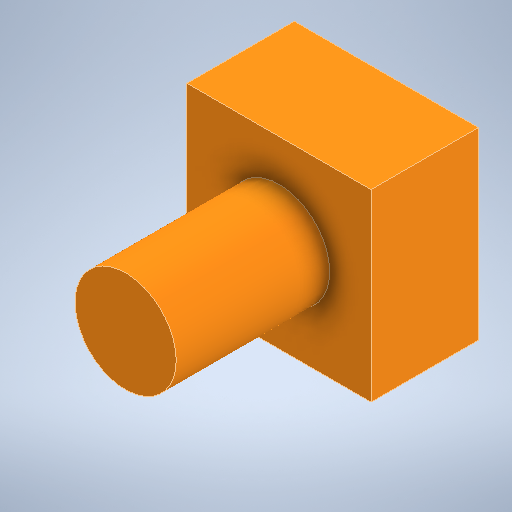
# Autodesk Inventor part: Button
Saved by Autodesk Inventor 2025.2 (Build 292293000, 293)
## iProperties
Created: 2025-04-06
Part Number: Button
Material: Generic
Document SubType Name: Modeling
Designer: eason
Density: 1 g/cm^3
Appearance: Orange
Author: eason
Autodesk Inventor part; units mm, degrees
ref_plane "YZ Plane" through (0, 0, 0) normal (1, 0, 0) x (0, 1, 0)
ref_plane "XZ Plane" through (0, 0, 0) normal (0, 1, 0) x (-1, 0, 0)
ref_plane "XY Plane" through (0, 0, 0) normal (0, 0, 1) x (1, 0, 0)
sketch "Sketch1" plane through (0, 0, 0) normal (0, 0, 1) x (1, 0, 0)
  circle A0 centre (0, 0) radius 1.65
  dimension "d0" = 3.3
  constraints: 1 centre point, 1 coincident
  measures "d0" diameter of A0
extrude "Extrusion1" add sketch "Sketch1" along normal blind 5
sketch "Sketch2" plane through (0, 0, 0) normal (0, 0, 1) x (1, 0, 0)
  line L0 (3, -3) -> (-3, -3)
  line L1 (-3, -3) -> (-3, 3)
  line L2 (-3, 3) -> (3, 3)
  line L3 (3, 3) -> (3, -3)
  line L4 (-4.2165, 0) -> (4.1835, 0) projected
  line L5 (0, -4.2) -> (0, 4.2) projected
  point P0 (0, 0)
  point P1 (3, 0)
  point P2 (0, 3)
  dimension "d3" = 6
  constraints: 8 end point, 2 midpoint, 2 parallel, 2 perpendicular, 2 point on line, 1 horizontal
  measures "d3" distance between parallel lines of L1 L3
extrude "Extrusion2" add sketch "Sketch2" against normal blind 3.5
body "Solid1"
